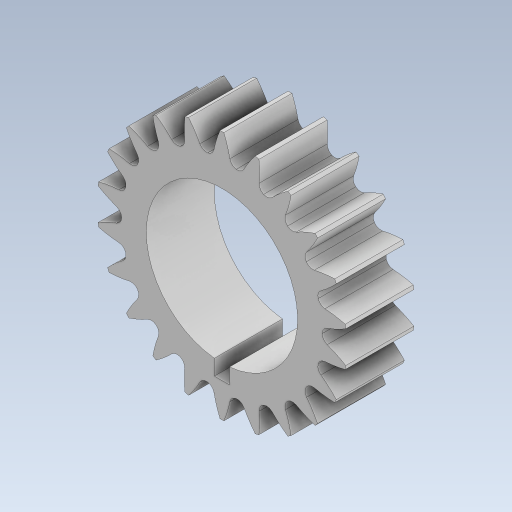
# Autodesk Inventor part: Pinion Lifter
Saved by Autodesk Inventor 2023.5 (Build 275446000, 446)
## iProperties
Created: 2025-09-02
Part Number: Pinion Lifter
Material: Generic
Document SubType Name: Modeling
Designer: Guntur
Density: 1 g/cm^3
Appearance: Default
Author: Guntur
Autodesk Inventor part; units mm, degrees
ref_plane "YZ Plane" through (0, 0, 0) normal (1, 0, 0) x (0, 1, 0)
ref_plane "XZ Plane" through (0, 0, 0) normal (0, 1, 0) x (-1, 0, 0)
ref_plane "XY Plane" through (0, 0, 0) normal (0, 0, 1) x (1, 0, 0)
sketch "Sketch1" plane through (0, 0, 0) normal (0, 0, 1) x (1, 0, 0)
  arc A0 (1, -9.9499) -> (-1, -9.9499) centre (0, 0) ccw
  line L0 (1, -11) -> (1, -9.9499)
  line L1 (-1, -11) -> (-1, -9.9499)
  circle A1 centre (0, 0) radius 15
  circle A2 centre (0, 0) radius 16.5
  circle A3 centre (0, 0) radius 13.25
  line L2 (0, 13.25) -> (0, 0) construction
  line L3 (0, 0) -> (-13.25, 0) construction
  line L4 (-1, -11) -> (-1, -12)
  line L5 (-1, -12) -> (1, -12)
  line L6 (1, -12) -> (1, -11)
  arc A4 (1.175, 13.1978) -> (0.25, 16.4981) centre (-12.6128, 11.1132) ccw
  arc A5 (-0.25, 16.4981) -> (-1.175, 13.1978) centre (12.6128, 11.1132) ccw
  point P0 (0.785, 14.9794)
  point P1 (-0.5, 16.4924)
  point P2 (-1.25, 13.1909)
  point P3 (-0.785, 14.9794)
  point P4 (-1.175, 13.1978)
  point P5 (-0.25, 16.4981)
  dimension "d0" = 20
  dimension "d3" = 30
  dimension "d4" = 33
  dimension "d5" = 26.5
  dimension "d17" = 1
  dimension "d20" = 1.57
  dimension "d23" = 2.35
  dimension "d24" = 0.5
  constraints: 15 point on circle, 14 end point, 6 centre point, 4 coincident, 3 perpendicular, 3 symmetric about line, 2 vertical, 1 horizontal alignment, 1 other
  measures "d0" diameter of A0
  measures "d3" diameter of A1
  measures "d4" diameter of A2
  measures "d5" diameter of A3
  measures "d17" distance of L1.start L4.end
  measures "d20" distance of A1.end A1.start
  measures "d23" distance of A5.end A4.start
  measures "d24" distance of A5.start A2.end
extrude "Extrusion3" add sketch "Sketch1" along normal blind 9 contours A3
extrude "Extrusion4" add sketch "Sketch1" along normal blind 9 contours A4 A3 A5 A1 | A1 A5 A2 A4 picked at (-0.0873, 13.8287) picked at (-0.0873, 15.6652)
fillet "Fillet2" radius 1 2 edges at (1.175, 13.1978, 4.5) (-1.175, 13.1978, 4.5)
pattern_circular "Circular Pattern1" count 22 over 360 about axis through (0, 0, -10) along (0, 0, 1) of "Extrusion4", "Fillet2"
body "Solid2"
